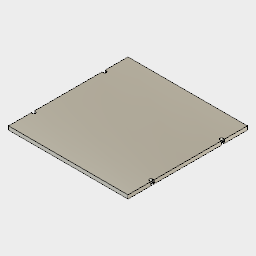
VORON2 Bed (Parametric) (Autodesk Fusion 360 design; units mm, degrees)
Autodesk Fusion 360 part; units mm, degrees
sketch "Sketch1" plane through (0, 0, 0) normal (0, 0, 1) x (1, 0, 0)
  line L0 (0, 0) -> (254, 0)
  line L1 (254, 0) -> (254, 254)
  line L2 (254, 254) -> (0, 254)
  line L3 (0, 254) -> (0, 0)
  line L4 (0, 127) -> (254, 127) construction
  line L5 (251, 200) -> (254, 200)
  line L6 (254, 204) -> (251, 204)
  arc A0 (251, 204) -> (251, 200) centre (251, 202) ccw
  line L7 (251, 202) -> (275, 202) construction
  line L8 (251, 50) -> (254, 50)
  line L9 (254, 54) -> (251, 54)
  arc A1 (251, 54) -> (251, 50) centre (251, 52) ccw
  line L10 (251, 52) -> (254, 52) construction
  line L11 (3, 204) -> (0, 204)
  line L12 (0, 200) -> (3, 200)
  arc A2 (3, 200) -> (3, 204) centre (3, 202) ccw
  line L13 (3, 202) -> (0, 202) construction
  line L14 (254, 205.25) -> (251, 205.25)
  arc A3 (251, 205.25) -> (251, 198.75) centre (251, 202) ccw
  line L15 (251, 198.75) -> (254, 198.75)
  line L16 (254, 55.25) -> (251, 55.25)
  arc A4 (251, 55.25) -> (251, 48.75) centre (251, 52) ccw
  line L17 (251, 48.75) -> (254, 48.75)
  line L18 (0, 198.75) -> (3, 198.75)
  arc A5 (3, 198.75) -> (3, 205.25) centre (3, 202) ccw
  line L19 (3, 205.25) -> (0, 205.25)
  line L20 (3, 54) -> (0, 54)
  line L21 (0, 50) -> (3, 50)
  arc A6 (3, 50) -> (3, 54) centre (3, 52) ccw
  line L22 (3, 52) -> (0, 52) construction
  line L23 (0, 48.75) -> (3, 48.75)
  arc A7 (3, 48.75) -> (3, 55.25) centre (3, 52) ccw
  line L24 (3, 55.25) -> (0, 55.25)
  point P0 (251, 202)
  point P1 (251, 52)
  point P2 (3, 52)
  point P3 (3, 202)
  dimension "d3" = 254
  dimension "d4" = 254
  dimension "d8" = 3
  dimension "d9" = 3
  dimension "d10" = 75
  dimension "d11" = 75
  dimension "d12" = 2
  dimension "d13" = 2
  dimension "d15" = 3
  dimension "d16" = 75
  dimension "d19" = 2
  dimension "d20" = 1.25
  dimension "d21" = 1.25
  dimension "d22" = 1.25
  dimension "d94" = 127
  dimension "d95" = 3
  dimension "d96" = 2
  dimension "d97" = 75
  dimension "d98" = 1.25
  measures "d3" distance of L0.start L0.end
  measures "d4" distance of L0.start L2.end
  measures "d8" distance of L1 P1
  measures "d9" distance of L1 P0
  measures "d10" distance of L4 P0
  measures "d11" distance of L4 P1
  measures "d12" radius of A1
  measures "d13" radius of A0
  measures "d15" distance of L3 P3
  measures "d16" distance of L4 P3
  measures "d19" radius of A2
  measures "d94" distance of L0 L4
  measures "d95" distance of L3 P2
  measures "d96" radius of A6
  measures "d97" distance of L4 P2
extrude "Extrude2" add sketch "Sketch1" along normal blind 4.95 contours L0 L1 L2 L3 L14 A3 L15 L16 A4 L17 L18 A5 L19 L23 A7 L24
extrude "Extrude3" add sketch "Sketch1" against normal blind 3 contours L0 L1 L2 L3 L14 A3 L15 L16 A4 L17 L18 A5 L19 L23 A7 L24 | L3 L20 L21 A6 L23 A7 L24 | L1 L8 L9 A1 L16 A4 L17 | L3 L11 L12 A2 L18 A5 L19 | L1 L5 L6 A0 L14 A3 L15
chamfer "Chamfer6" distance 0.5 angle 45 16 edges at (0, 205.25, 2.475) (0, 198.75, 2.475) (0, 204, -1.5) (0, 200, -1.5) (0, 55.25, 2.475) (0, 48.75, 2.475) (0, 50, -1.5) (0, 54, -1.5) (254, 48.75, 2.475) (254, 55.25, 2.475) (254, 54, -1.5) (254, 50, -1.5) (254, 205.25, 2.475) (254, 198.75, 2.475) (254, 200, -1.5) (254, 204, -1.5)
equation "x_bed_size = 10 in"
equation "y_bed_size = 10 in"
equation "d3 = x_bed_size"
equation "d4 = y_bed_size"
equation "d8 = d9"
equation "d10 = ( 150 / 2 ) * 1 mm"
equation "d11 = d10"
equation "d12 = d13"
equation "d15 = d9"
equation "d16 = d10"
equation "d19 = d13"
equation "d21 = d20"
equation "d22 = d20"
equation "d23 = 7.95 mm - 3 mm"
equation "d94 = y_bed_size / 2"
equation "d95 = d15"
equation "d96 = d19"
equation "d97 = d16"
